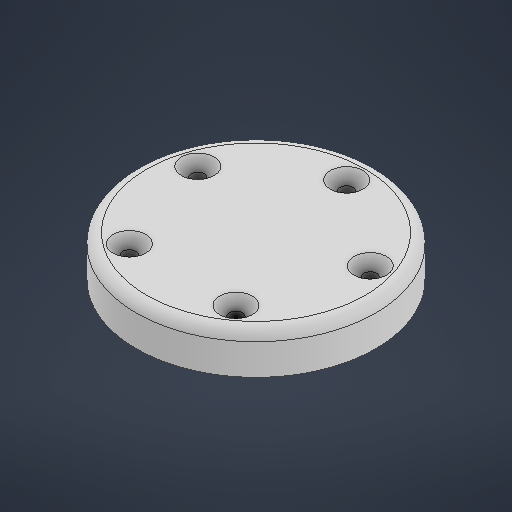
# Autodesk Inventor part: bearingplate
Saved by Autodesk Inventor 2026 (Build 300175000, 175)
## iProperties
Created: 2026-04-21
Part Number: bearingplate
Material: Generic
Document SubType Name: Modeling
Designer: oleg2
Density: 1 g/cm^3
Appearance: Default
Author: oleg2
Autodesk Inventor part; units mm, degrees
ref_plane "YZ Plane" through (0, 0, 0) normal (1, 0, 0) x (0, 1, 0)
ref_plane "XZ Plane" through (0, 0, 0) normal (0, 1, 0) x (-1, 0, 0)
ref_plane "XY Plane" through (0, 0, 0) normal (0, 0, 1) x (1, 0, 0)
sketch "Sketch1" plane through (0, 0, 0) normal (0, 1, 0) x (-1, 0, 0)
  circle A0 centre (0, 0) radius 36.83
  dimension "d0" = 73.66
  constraints: 1 centre point, 1 coincident
  measures "d0" diameter of A0
extrude "Extrusion1" add sketch "Sketch1" along normal blind 12.7
fillet "Fillet1" radius 3.175 1 edges at (36.83, 12.7, 0)
sketch "Sketch3" plane through (0, 0, 0) normal (0, -1, 0) x (1, 0, 0)
  circle A0 centre (0, 0) radius 19.05
  dimension "d12" = 38.1
  constraints: 1 centre point, 1 coincident
  measures "d12" diameter of A0
extrude "Extrusion3" cut sketch "Sketch3" against normal blind 6.35
chamfer "Chamfer1" distance 3.175 angle 45 2 edges at (-19.05, 0, 0) (-19.05, 6.35, 0)
sketch "Sketch5" plane through (0, 12.7, 0) normal (0, 1, 0) x (1, 0, 0)
  line L0 (0, 0) -> (0, 27.94)
  point P0 (-26.5725, 8.6339)
  point P1 (-26.5725, 8.6339)
  point P2 (-16.4227, -22.6039)
  point P3 (-16.4227, -22.6039)
  point P4 (16.4227, -22.6039)
  point P5 (16.4227, -22.6039)
  point P6 (26.5725, 8.6339)
  point P7 (26.5725, 8.6339)
  dimension "d18" = 27.94
  dimension "d21" = 360
  constraints: 5 coincident, 2 end point, 1 vertical, 11 other
  measures "d18" distance of L0.start L0.end
hole "Hole1" at (0, 12.7, -27.94) at (-26.5725, 12.7, -8.6339) at (-16.4227, 12.7, 22.6039) at (16.4227, 12.7, 22.6039) at (26.5725, 12.7, -8.6339) direction (0, -1, 0) diameter 4 end through all countersink diameter 10 countersink angle 90
body "Solid1"
